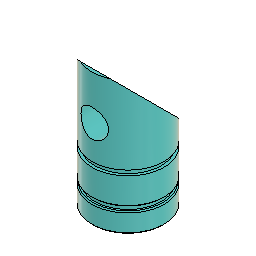
SUPPORT_POINTEUR_AIR_ASSIST v15 (Autodesk Fusion 360 archive; units mm, degrees)
design "LASER_K40_HEAD"
Autodesk Fusion 360 part; units mm, degrees
note: some values were not read from the file. Chosen so that the rebuilt part matches the saved one: which face or edge a step refers to. Set by a fixed rule: which sketch regions a step uses.
sketch "Sketch1" plane through (0, 0, 0) normal (0, 0, 1) x (1, 0, 0)
  circle A0 centre (0, 0) radius 13
  circle A1 centre (0, 0) radius 12
  dimension "d1" = 26
  dimension "d2" = 24
  constraint coincident A0.centre A1.centre
  constraint concentric A0 A1
  measures "d1" diameter of A0
  measures "d2" diameter of A1
extrude "Extrude1" add sketch "Sketch1" along normal blind 7 contours A0 | A1
extrude "Extrude2" add sketch "Sketch1" along normal blind 8.518 contours A1
sketch "Sketch2" plane through (0, 0, 8.518) normal (0, 0, 1) x (-1, 0, 0)
  circle A0 centre (0, 0) radius 12
  circle A1 centre (0, 0) radius 13
  circle A2 centre (0, 0) radius 13
  constraint coincident A0.centre A1.centre
  constraint tangent A1 A2
extrude "Extrude4" add sketch "Sketch2" along normal blind 9.701 contours A0 | A1 A2
chamfer "Chamfer1" distance 0.4 angle 45 1 edges at (-12.1203, -4.701, 0)
chamfer "Chamfer2" distance 0.4 angle 45 2 edges at (12.1203, 4.701, 8.518) (-12.1203, -4.701, 7)
sketch "Sketch3" plane through (0, 0, 18.219) normal (0, 0, 1) x (-1, 0, 0)
  circle A0 centre (0, 0) radius 13
  circle A1 centre (0, 0) radius 12
  dimension "d14" = 24
  constraint coincident A0.centre A1.centre
  measures "d14" diameter of A1
extrude "Extrude5" add sketch "Sketch3" along normal blind 1.8 contours A1
sketch "Sketch4" plane through (0, 0, 20.019) normal (0, 0, 1) x (-1, 0, 0)
  circle A0 centre (0, 0) radius 12
  circle A1 centre (0, 0) radius 13
  dimension "d17" = 26
  constraint coincident A0.centre A1.centre
  measures "d17" diameter of A1
extrude "Extrude6" add sketch "Sketch4" along normal blind 28 contours A0 | A1
sketch "Sketch5" plane through (0, 0, 0) normal (1, 0, 0) x (0, 1, 0)
  line L0 (-11.8, 48.019) -> (13, 23.219)
  line L1 (13, 48.019) -> (-13, 48.019)
  line L2 (13, 48.019) -> (13, 23.219)
  line L3 (13, 20.019) -> (-13, 20.019) construction
  dimension "d20" = 45
  dimension "d21" = 3.2
  constraint coincident L0.start L1
  constraint coincident L1.start L2.start
  constraint vertical L2
  measures "d20" angle of L0 L2
  measures "d21" distance of L0.end L3.start
extrude "Extrude7" cut sketch "Sketch5" along normal through all and the other way through all
ref_plane "WorkPlane1" through (0, -13, 37.2678) normal (0, -1, 0) x (-1, 0, 0)
sketch "Sketch6" plane through (0, -13, 37.2678) normal (0, -1, 0) x (1, 0, 0)
  line L0 (13, -17.2488) -> (-13, -17.2488)
  line L1 (0, -17.2488) -> (0, -5.2488) construction
  circle A0 centre (0, -5.2488) radius 5
  dimension "d24" = 12
  dimension "d25" = 10
  constraint midpoint L0 L1.start
  constraint perpendicular L0 L1
  constraint coincident L1.end A0.centre
  measures "d24" distance of L1.start L1.end
  measures "d25" diameter of A0
extrude "Extrude8" cut sketch "Sketch6" against normal blind 8.188

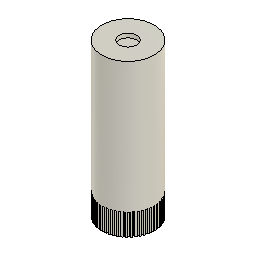
design "POINTEUR_SYD1230"
Autodesk Fusion 360 part; units mm, degrees
sketch "Sketch1" plane through (0, 0, 0) normal (0, 0, 1) x (1, 0, 0)
  circle A0 centre (0, 0) radius 6
  dimension "d1" = 12
  constraint coincident A0.centre origin
  measures "d1" diameter of A0
extrude "Extrude1" add sketch "Sketch1" along normal blind 35
sketch "Sketch2" plane through (0, 0, 35) normal (0, 0, 1) x (-1, 0, 0)
  circle A0 centre (0, 0) radius 6
  circle A1 centre (0, 0) radius 1.9846
  constraint coincident A0.centre A1.centre
extrude "Extrude2" cut sketch "Sketch2" against normal blind 0.967 contours A1
sketch "Sketch3" plane through (0, 0, 0) normal (0, 0, -1) x (1, 0, 0)
  circle A0 centre (0, 0) radius 6
  circle A1 centre (0, 0) radius 3.5
  dimension "d6" = 7
  constraint coincident A0.centre A1.centre
  measures "d6" diameter of A1
extrude "Extrude3" cut sketch "Sketch3" against normal blind 0.666 contours A1
sketch "Sketch4" plane through (0, 0, 0) normal (0, 0, -1) x (1, 0, 0)
  circle A0 centre (0, 0) radius 3.5
  circle A1 centre (0, 0) radius 6
  line L0 (6.1415, 0.289) -> (6.1124, 0.289)
  line L1 (6.1124, 0.289) -> (5.664, -0.0017)
  line L2 (5.664, -0.0017) -> (6.1913, -0.2425)
  line L3 (6.1913, -0.2425) -> (6.1415, 0.289)
  constraint horizontal L0
extrude "Extrude4" cut sketch "Sketch4" against normal blind 5 contours A1 L1 L2 picked at (5.8879, 0.0232)
pattern_circular "C-Pattern1" count 50 over 360 about axis through (0, 0, 0) along (0, 0, 1) of "Extrude4"

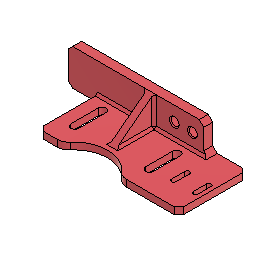
design "SUPPORT_DRAG_CHAINE"
Autodesk Fusion 360 part; units mm, degrees
sketch "Sketch1" plane through (0, 0, 0) normal (0, 0, 1) x (1, 0, 0)
  circle A0 centre (0, 0) radius 15
  line L0 (-18.25, 29) -> (-18.25, 17)
  arc A1 (-18.25, 17) -> (-14.75, 17) centre (-16.5, 17) ccw
  line L1 (-14.75, 17) -> (-14.75, 29)
  arc A2 (-14.75, 29) -> (-18.25, 29) centre (-16.5, 29) ccw
  line L2 (-16.5, 29) -> (-16.5, 17) construction
  circle A3 centre (0, 0) radius 13 construction
  line L3 (-12.6886, 8) -> (-23.5, 8)
  line L4 (-23.5, 8) -> (-23.5, 38)
  line L5 (-23.5, 38) -> (0, 38)
  line L6 (-23.5, 34) -> (0, 34)
  line L7 (0, 0) -> (0, 38) construction
  line L8 (-23.5, 34) -> (-36.5, 34)
  line L9 (-36.5, 34) -> (-36.5, 38)
  line L10 (-36.5, 38) -> (-23.5, 38)
  line L11 (12.6886, 8) -> (23.5, 8)
  line L12 (23.5, 8) -> (23.5, 38) construction
  line L13 (14.75, 17) -> (14.75, 29)
  arc A4 (18.25, 29) -> (14.75, 29) centre (16.5, 29) ccw
  arc A5 (14.75, 17) -> (18.25, 17) centre (16.5, 17) ccw
  line L14 (18.25, 29) -> (18.25, 17)
  line L15 (23.5, 34) -> (0, 34)
  line L16 (23.5, 38) -> (0, 38)
  line L17 (23.5, 8) -> (38.5, 8)
  line L18 (38.5, 8) -> (38.5, 34)
  line L19 (38.5, 34) -> (23.5, 34)
  line L20 (23.5, 38) -> (23.5, 34)
  line L21 (25.2, 24) -> (25.2, 18)
  arc A6 (25.2, 18) -> (27.2, 18) centre (26.2, 18) ccw
  line L22 (27.2, 18) -> (27.2, 24)
  arc A7 (27.2, 24) -> (25.2, 24) centre (26.2, 24) ccw
  line L23 (26.2, 24) -> (26.2, 18) construction
  line L24 (31, 34) -> (31, 8) construction
  line L25 (26.2, 21) -> (31, 21) construction
  line L26 (36.8, 24) -> (36.8, 18)
  arc A8 (34.8, 18) -> (36.8, 18) centre (35.8, 18) ccw
  line L27 (34.8, 18) -> (34.8, 24)
  arc A9 (36.8, 24) -> (34.8, 24) centre (35.8, 24) ccw
  line L28 (23.5, 38) -> (38.5, 38)
  line L29 (38.5, 38) -> (38.5, 34)
  dimension "d1" = 30
  dimension "d2" = 16.5
  dimension "d3" = 1.75
  dimension "d4" = 12
  dimension "d5" = 29
  dimension "d6" = 26
  dimension "d7" = 8
  dimension "d9" = 4
  dimension "d10" = 5
  dimension "d11" = 23.5
  dimension "d12" = 60
  dimension "d13" = 15
  dimension "d14" = 3.8
  dimension "d15" = 1
  dimension "d16" = 6
  constraint tangent L0 A1
  constraint tangent A1 L1
  constraint parallel L0 L1
  constraint tangent L1 A2
  constraint tangent L0 A2
  constraint vertical L2
  constraint concentric A0 A3
  constraint coincident A0 L3.start
  constraint perpendicular L1 L3
  constraint perpendicular L3 L4
  constraint perpendicular L4 L5
  constraint coincident L4 L6.start
  constraint perpendicular L4 L6
  constraint coincident A0.centre A3.centre
  constraint perpendicular L5 L7
  constraint coincident L6.end L7
  constraint perpendicular L4 L8
  constraint perpendicular L8 L9
  constraint horizontal L10
  constraint symmetric L0.start L7 A4.start
  constraint symmetric L0.end L7 A5.end
  constraint symmetric A1.end L7 L13.start
  constraint symmetric L1.end L7 L13.end
  constraint symmetric A1 L7 A5
  constraint symmetric A2 L7 A4
  constraint symmetric L3.start L7 L11.start
  constraint symmetric L3.end L7 L11.end
  constraint symmetric L4.end L7 L12.end
  constraint symmetric L5.end L7 L16.end
  constraint symmetric L6.start L7 L15.start
  constraint symmetric L6.end L7 L15.end
  constraint perpendicular L12 L17
  constraint perpendicular L17 L18
  constraint horizontal L19
  constraint tangent L21 A6
  constraint tangent A6 L22
  constraint parallel L21 L22
  constraint tangent L22 A7
  constraint tangent L21 A7
  constraint perpendicular L6 L23
  constraint midpoint L19 L24.start
  constraint midpoint L17 L24.end
  constraint midpoint L23 L25.start
  constraint midpoint L24 L25.end
  constraint horizontal L25
  constraint symmetric L21.start L24 L26.start
  constraint symmetric L21.end L24 L26.end
  constraint symmetric A6.end L24 A8.start
  constraint symmetric L22.end L24 L27.end
  constraint symmetric A6 L24 A8
  constraint symmetric A7 L24 A9
  constraint perpendicular L12 L28
  constraint vertical L29
  measures "d1" diameter of A0
  measures "d2" distance of A0.centre L2
  measures "d3" radius of A1
  measures "d4" distance of A2.centre A1.centre
  measures "d5" vertical distance of A0.centre A2.centre
  measures "d6" diameter of A3
  measures "d7" distance of A0.centre L3
  measures "d9" distance of L5 L6
  measures "d10" distance of A2.centre L6
  measures "d11" distance of A0.centre L4
  measures "d12" distance of L9 L12
  measures "d13" distance of L12 L18
  measures "d14" distance of L22 L24
  measures "d15" radius of A7
  measures "d16" distance of A7.centre A6.centre
extrude "Extrude1" add sketch "Sketch1" along normal blind 3 contours A0 L3 L4 L6 L11 L15 L17 L18 L19 | L19 L20 L28 L29
extrude "Extrude2" add sketch "Sketch1" along normal blind 16 contours L4 L8 L9 L10 | L4 L5 L6 L15 L16 L20
chamfer "Chamfer1" distance 2 angle 45 1 edges at (23.5, 36, 3)
chamfer "Chamfer2" distance 2 angle 45 3 edges at (38.5, 38, 1.5) (38.5, 8, 1.5) (-23.5, 8, 1.5)
fillet "Fillet1" radius 5 2 edges at (-12.6886, 8, 1.5) (12.6886, 8, 1.5)
sketch "Sketch2" plane through (0, 0, 0) normal (1, 0, 0) x (0, 1, 0)
  line L0 (34, 3) -> (34, 5)
  line L1 (34, 5) -> (34, 16)
  line L2 (34, 16) -> (34, 0)
  line L3 (34, 0) -> (34, 3)
  line L4 (8, 3) -> (9.75, 3)
  line L5 (8, 3) -> (10, 3)
  line L6 (10, 3) -> (36, 3)
  line L7 (36, 3) -> (38, 3)
  line L8 (38, 3) -> (34, 3)
  line L9 (34, 3) -> (10, 3)
  line L10 (10, 3) -> (8, 3)
  line L11 (8, 3) -> (9.75, 3)
  line L12 (9.75, 3) -> (15, 3)
  line L13 (29, 3) -> (17, 3)
  line L14 (15.25, 3) -> (17, 3)
  line L15 (17, 3) -> (29, 3)
  line L16 (29, 3) -> (30.75, 3)
  line L17 (17, 3) -> (29, 3)
  line L18 (29, 3) -> (30.75, 3)
  line L19 (29, 3) -> (17, 3)
  line L20 (15.25, 3) -> (17, 3)
  line L21 (24, 3) -> (18, 3)
  line L22 (17, 3) -> (18, 3)
  line L23 (18, 3) -> (24, 3)
  line L24 (24, 3) -> (25, 3)
  line L25 (18, 3) -> (24, 3)
  line L26 (24, 3) -> (25, 3)
  line L27 (24, 3) -> (18, 3)
  line L28 (17, 3) -> (18, 3)
  line L29 (34, 16) -> (17, 3)
  constraint coincident L1.end L2.start
  constraint coincident L13.end L14.end
extrude "Extrude3" add sketch "Sketch2" along normal mid plane 3
chamfer "Chamfer3" distance 1 angle 45 6 edges at (1.5, 34, 9.5) (-1.5, 34, 9.5) (-1.5, 25.5, 3) (-12.5, 34, 3) (13.5, 34, 3) (1.5, 25.5, 3)
sketch "Sketch3" plane through (0, 38, 0) normal (0, 1, 0) x (-1, 0, 0)
  line L0 (-36.5, 3) -> (-36.5, 0)
  line L1 (-36.5, 0) -> (36.5, 0)
  line L2 (36.5, 0) -> (36.5, 16)
  line L3 (36.5, 16) -> (-23.5, 16)
  line L4 (-23.5, 16) -> (-23.5, 5)
  line L5 (-23.5, 5) -> (-25.5, 3)
  line L6 (-25.5, 3) -> (-36.5, 3)
  line L7 (36.5, 9.5) -> (-23.5, 9.5) construction
  circle A0 centre (-18.5, 9.5) radius 1.75
  circle A1 centre (-10.5, 9.5) radius 1.75
  dimension "d27" = 6.5
  dimension "d28" = 3.5
  dimension "d29" = 8
  dimension "d30" = 5
  constraint coincident L2 L7.start
  constraint coincident L4 L7.end
  constraint horizontal L7
  constraint coincident L7 A0.centre
  constraint coincident L7 A1.centre
  constraint equal A0 A1
  measures "d27" distance of L3 L7
  measures "d28" diameter of A0
  measures "d29" distance of A0.centre A1.centre
  measures "d30" distance of L4 A0.centre
extrude "Extrude4" cut sketch "Sketch3" against normal through all contours A0 | A1
chamfer "Chamfer4" distance 0.4 angle 45 4 edges at (20.1316, 38, 10.1328) (12.1316, 38, 10.1328) (20.1316, 34, 8.8672) (12.1316, 34, 8.8672)
chamfer "Chamfer5" distance 2 angle 45 1 edges at (23.5, 36, 16)
chamfer "Chamfer6" distance 2 angle 45 2 edges at (-36.5, 36, 0) (-36.5, 36, 16)
equation "d2 = ( 33 / 2 ) * 1 mm"
equation "d3 = ( 3.5 / 2 ) * 1 mm"
equation "d11 = ( 47 / 2 ) * 1 mm"
equation "d19 = 13 mm + 3 mm"
